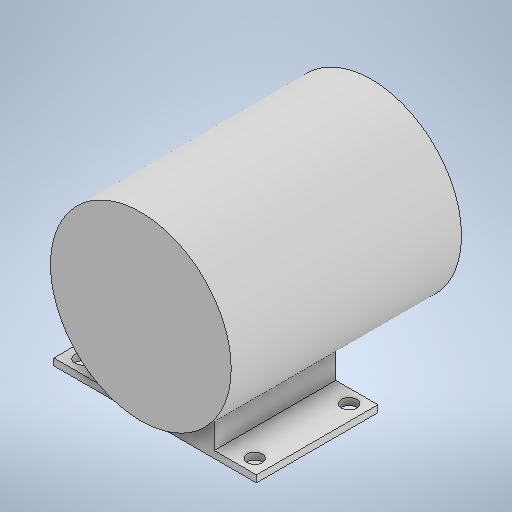
# Autodesk Inventor part: BLDC BM1109 MOTOR
Saved by Autodesk Inventor 2025.2 (Build 292293000, 293)
## iProperties
Created: 2025-03-19
Part Number: BLDC BM1109 MOTOR
Material: Generic
Document SubType Name: Modeling
Designer: Mathias B. Kampp
Density: 1 g/cm^3
Appearance: Default
Author: Mathias B. Kampp
Autodesk Inventor part; units mm, degrees
ref_plane "YZ Plane" through (0, 0, 0) normal (1, 0, 0) x (0, 1, 0)
ref_plane "XZ Plane" through (0, 0, 0) normal (0, 1, 0) x (-1, 0, 0)
ref_plane "XY Plane" through (0, 0, 0) normal (0, 0, 1) x (1, 0, 0)
sketch "Sketch1" plane through (0, 0, 0) normal (0, 1, 0) x (-1, 0, 0)
  line L0 (0, 0) -> (-120, 0)
  line L1 (-120, 0) -> (-120, -72)
  line L2 (-120, -72) -> (0, -72)
  line L3 (0, -72) -> (0, 0)
  circle A0 centre (-9, -8) radius 4.5
  circle A1 centre (-111, -8) radius 4.5
  circle A2 centre (-9, -64) radius 4.5
  circle A3 centre (-111, -64) radius 4.5
  dimension "d0" = 120
  dimension "d1" = 72
  dimension "d2" = 9
  dimension "d3" = 9
  dimension "d4" = 9
  dimension "d5" = 9
  constraints: 8 end point, 4 centre point, 2 parallel, 1 horizontal, 1 perpendicular
  measures "d0" distance of L2.end L1.end
  measures "d1" distance of L1.end L0.end
  measures "d2" diameter of A0
  measures "d3" diameter of A1
  measures "d4" diameter of A2
  measures "d5" diameter of A3
extrude "Extrusion1" add sketch "Sketch1" along normal blind 4.1
sketch "Sketch2" plane through (0, 4.1, 0) normal (0, 1, 0) x (1, 0, 0)
  line L0 (0, 0) -> (120, 0) projected
  line L1 (120, 72) -> (0, 72) projected
  line L2 (25, 0) -> (95, 0)
  line L3 (95, 0) -> (95, 72)
  line L4 (95, 72) -> (25, 72)
  line L5 (25, 72) -> (25, 0)
  dimension "d8" = 70
  constraints: 8 end point, 2 parallel, 2 point on line, 1 horizontal, 1 perpendicular
  measures "d8" distance of L4.end L3.end
extrude "Extrusion2" add sketch "Sketch2" along normal blind 53.5
sketch "Sketch3" plane through (0, 0, 0) normal (0, 0, 1) x (1, 0, 0)
  circle A0 centre (60, 59.6) radius 53.5
  point P0 (0, 0)
  dimension "d11" = 107
  constraints: 1 centre point
  measures "d11" diameter of A0
extrude "Extrusion3" add sketch "Sketch3" along normal blind 8.5 and the other way blind 128
body "Solid1"
